Autodesk Inventor part; units mm, degrees
(part 13 of 16)
  spline S79 degree 3 poles (53.7291, 72.5452) (53.576, 72.5257) (53.422, 72.5132) (53.2678, 72.5092) (53.222, 72.508) (53.1761, 72.5076) (53.1303, 72.5079) (53.0872, 72.5083) (53.0441, 72.5093) (53.001, 72.5111) (52.9608, 72.5127) (52.9205, 72.515) (52.8803, 72.518) (52.8429, 72.5208) (52.8055, 72.5243) (52.7682, 72.5283) (52.7337, 72.5321) (52.6992, 72.5364) (52.6648, 72.5413) (52.6332, 72.5458) (52.6016, 72.5509) (52.5701, 72.5565) (52.5414, 72.5616) (52.5127, 72.5671) (52.4842, 72.5732) (52.4584, 72.5787) (52.4327, 72.5846) (52.407, 72.5909) (52.384, 72.5965) (52.3611, 72.6024) (52.3385, 72.6091) (52.3186, 72.615) (52.2989, 72.6215) (52.2786, 72.6272) (52.2408, 72.6377) (52.2006, 72.6455) (52.1693, 72.667) (52.1455, 72.6832) (52.1269, 72.7073) (52.1064, 72.7287) (52.0892, 72.7466) (52.0706, 72.7625) (52.0521, 72.7786) (52.034, 72.7943) (52.016, 72.8102) (51.9977, 72.8256) (51.9798, 72.8407) (51.9617, 72.8554) (51.9433, 72.8698) (51.9254, 72.8839) (51.9073, 72.8977) (51.889, 72.9112) (51.8711, 72.9244) (51.8531, 72.9372) (51.8348, 72.9498) (51.8169, 72.962) (51.7989, 72.974) (51.7806, 72.9856) (51.7628, 72.9969) (51.7448, 73.0079) (51.7266, 73.0186) (51.7088, 73.029) (51.6909, 73.0391) (51.6727, 73.0489) (51.655, 73.0584) (51.6371, 73.0676) (51.619, 73.0764) (51.6013, 73.085) (51.5834, 73.0933) (51.5653, 73.1012) (51.5476, 73.1089) (51.5298, 73.1162) (51.5118, 73.1232) (51.4941, 73.13) (51.4762, 73.1364) (51.4582, 73.1424) (51.4405, 73.1483) (51.4226, 73.1538) (51.4046, 73.1588) (51.3868, 73.1638) (51.3689, 73.1683) (51.3509, 73.1724) (51.333, 73.1763) (51.315, 73.1799) (51.297, 73.1828) (51.2789, 73.1858) (51.2608, 73.1882) (51.2427, 73.1901) (51.2244, 73.192) (51.2062, 73.1933) (51.1879, 73.194) (51.1694, 73.1947) (51.151, 73.1947) (51.1325, 73.1941) (51.1138, 73.1935) (51.0951, 73.1922) (51.0765, 73.1901) (51.0575, 73.188) (51.0386, 73.1851) (51.0198, 73.1815) (51.0005, 73.1777) (50.9814, 73.173) (50.9626, 73.1675) (50.9431, 73.1618) (50.924, 73.1552) (50.9052, 73.1477) (50.8858, 73.1398) (50.8667, 73.131) (50.8483, 73.1211) (50.8291, 73.111) (50.8106, 73.0997) (50.7928, 73.0874) (50.7744, 73.0748) (50.7567, 73.061) (50.74, 73.0462) (50.7229, 73.0311) (50.7068, 73.0148) (50.6916, 72.9977) (50.6808, 72.9856) (50.6705, 72.973) (50.6603, 72.9603) (50.6116, 72.8993) (50.5669, 72.8352) (50.5184, 72.7741) (50.4699, 72.713) (50.4176, 72.6548) (50.3693, 72.5935) (50.3592, 72.5808) (50.3493, 72.5679) (50.3399, 72.5546) (50.3267, 72.5359) (50.3146, 72.5165) (50.3037, 72.4964) (50.2931, 72.4768) (50.2837, 72.4565) (50.2755, 72.4357) (50.2676, 72.4155) (50.2609, 72.3949) (50.2553, 72.374) (50.2499, 72.3538) (50.2456, 72.3332) (50.2424, 72.3125) (50.2393, 72.2925) (50.2372, 72.2724) (50.2361, 72.2521) (50.235, 72.2325) (50.2348, 72.2129) (50.2355, 72.1933) (50.2362, 72.1741) (50.2377, 72.1551) (50.24, 72.1361) (50.2422, 72.1175) (50.2451, 72.099) (50.2488, 72.0806) (50.2524, 72.0625) (50.2566, 72.0445) (50.2615, 72.0267) (50.2663, 72.0091) (50.2717, 71.9916) (50.2777, 71.9742) (50.2836, 71.957) (50.2901, 71.9399) (50.2971, 71.923) (50.3041, 71.9061) (50.3116, 71.8894) (50.3196, 71.8729) (50.3276, 71.8562) (50.336, 71.8398) (50.3449, 71.8236) (50.3539, 71.8072) (50.3633, 71.7911) (50.3731, 71.7751) (50.383, 71.759) (50.3933, 71.7431) (50.404, 71.7274) (50.4148, 71.7114) (50.426, 71.6957) (50.4376, 71.6802) (50.4494, 71.6644) (50.4615, 71.6489) (50.4739, 71.6336) (50.4866, 71.618) (50.4996, 71.6026) (50.5129, 71.5875) (50.5265, 71.572) (50.5404, 71.5568) (50.5546, 71.5419) (50.5692, 71.5266) (50.584, 71.5115) (50.5991, 71.4968) (50.6145, 71.4816) (50.6302, 71.4668) (50.6462, 71.4522) (50.6626, 71.4372) (50.6792, 71.4225) (50.6961, 71.4081) (50.7134, 71.3933) (50.7309, 71.3788) (50.7487, 71.3646) (50.7669, 71.35) (50.7854, 71.3357) (50.8041, 71.3217) (50.8233, 71.3074) (50.8429, 71.2935) (50.8623, 71.2794) (50.8821, 71.2651) (50.9019, 71.2506) (50.9232, 71.2379) (50.9486, 71.2227) (50.9764, 71.2101) (50.9976, 71.1907) (51.0256, 71.165) (51.0423, 71.1276) (51.0612, 71.0932) (51.0713, 71.0747) (51.0821, 71.0571) (51.0924, 71.039) (51.104, 71.0185) (51.1149, 70.9975) (51.1256, 70.9764) (51.1376, 70.9528) (51.1492, 70.9291) (51.1604, 70.9052) (51.1728, 70.8788) (51.1847, 70.8522) (51.1962, 70.8253) (51.2088, 70.796) (51.2209, 70.7664) (51.2325, 70.7366) (51.2451, 70.7042) (51.2571, 70.6716) (51.2686, 70.6388) (51.2811, 70.6034) (51.2929, 70.5678) (51.3041, 70.532) (51.3162, 70.4935) (51.3275, 70.4548) (51.3383, 70.416) (51.3498, 70.3745) (51.3606, 70.3328) (51.3707, 70.2909) (51.3814, 70.2463) (51.3914, 70.2015) (51.4007, 70.1566) (51.4318, 70.0055) (51.4546, 69.8527) (51.4704, 69.6993) knots 0 0 0 0 0.065113 0.065113 0.065113 0.084473 0.084473 0.084473 0.102659 0.102659 0.102659 0.119672 0.119672 0.119672 0.135512 0.135512 0.135512 0.150178 0.150178 0.150178 0.163672 0.163672 0.163672 0.175991 0.175991 0.175991 0.187138 0.187138 0.187138 0.197111 0.197111 0.197111 0.205911 0.205911 0.205911 0.222284 0.222284 0.222284 0.234681 0.234681 0.234681 0.24506 0.24506 0.24506 0.255176 0.255176 0.255176 0.265035 0.265035 0.265035 0.274643 0.274643 0.274643 0.284008 0.284008 0.284008 0.293139 0.293139 0.293139 0.302047 0.302047 0.302047 0.310743 0.310743 0.310743 0.319241 0.319241 0.319241 0.327556 0.327556 0.327556 0.335706 0.335706 0.335706 0.343713 0.343713 0.343713 0.351599 0.351599 0.351599 0.359392 0.359392 0.359392 0.367126 0.367126 0.367126 0.374835 0.374835 0.374835 0.382562 0.382562 0.382562 0.390352 0.390352 0.390352 0.398256 0.398256 0.398256 0.406325 0.406325 0.406325 0.41461 0.41461 0.41461 0.423156 0.423156 0.423156 0.431994 0.431994 0.431994 0.441132 0.441132 0.441132 0.450548 0.450548 0.450548 0.460189 0.460189 0.460189 0.467051 0.467051 0.467051 0.5 0.5 0.5 0.532949 0.532949 0.532949 0.539811 0.539811 0.539811 0.549452 0.549452 0.549452 0.558868 0.558868 0.558868 0.568006 0.568006 0.568006 0.576844 0.576844 0.576844 0.58539 0.58539 0.58539 0.593675 0.593675 0.593675 0.601744 0.601744 0.601744 0.609648 0.609648 0.609648 0.617438 0.617438 0.617438 0.625165 0.625165 0.625165 0.632874 0.632874 0.632874 0.640608 0.640608 0.640608 0.648401 0.648401 0.648401 0.656287 0.656287 0.656287 0.664294 0.664294 0.664294 0.672444 0.672444 0.672444 0.680759 0.680759 0.680759 0.689257 0.689257 0.689257 0.697953 0.697953 0.697953 0.706861 0.706861 0.706861 0.715992 0.715992 0.715992 0.725357 0.725357 0.725357 0.734965 0.734965 0.734965 0.744824 0.744824 0.744824 0.75494 0.75494 0.75494 0.765319 0.765319 0.765319 0.777716 0.777716 0.777716 0.794089 0.794089 0.794089 0.802889 0.802889 0.802889 0.812862 0.812862 0.812862 0.824009 0.824009 0.824009 0.836328 0.836328 0.836328 0.849822 0.849822 0.849822 0.864488 0.864488 0.864488 0.880328 0.880328 0.880328 0.897341 0.897341 0.897341 0.915527 0.915527 0.915527 0.934887 0.934887 0.934887 1 1 1 1
  arc A282 (53.7291, 72.5452) -> (54.1249, 73.4583) centre (45.7832, 76.5321) ccw
  spline S80 degree 3 poles (54.658, 77.0523) (54.5352, 76.9589) (54.4081, 76.8711) (54.2766, 76.7905) (54.2374, 76.7665) (54.1979, 76.7432) (54.1581, 76.7206) (54.1206, 76.6993) (54.0828, 76.6787) (54.0446, 76.6587) (54.0089, 76.64) (53.9729, 76.6219) (53.9366, 76.6044) (53.9027, 76.5881) (53.8687, 76.5724) (53.8343, 76.5572) (53.8025, 76.5432) (53.7705, 76.5297) (53.7383, 76.5168) (53.7086, 76.5049) (53.6787, 76.4935) (53.6487, 76.4826) (53.6213, 76.4726) (53.5937, 76.4631) (53.5659, 76.4541) (53.5408, 76.4459) (53.5156, 76.4382) (53.4902, 76.4308) (53.4675, 76.4242) (53.4446, 76.4178) (53.4218, 76.4123) (53.4016, 76.4075) (53.3813, 76.4033) (53.3609, 76.398) (53.3228, 76.3883) (53.2841, 76.3749) (53.2463, 76.3778) (53.2176, 76.3801) (53.1894, 76.3916) (53.161, 76.3998) (53.1371, 76.4067) (53.1131, 76.4112) (53.089, 76.4159) (53.0655, 76.4205) (53.042, 76.4252) (53.0184, 76.4295) (52.9954, 76.4336) (52.9723, 76.4372) (52.9492, 76.4406) (52.9267, 76.4438) (52.9041, 76.4467) (52.8815, 76.4492) (52.8594, 76.4517) (52.8373, 76.4538) (52.8152, 76.4555) (52.7936, 76.4572) (52.772, 76.4585) (52.7504, 76.4594) (52.7293, 76.4603) (52.7082, 76.4609) (52.6871, 76.461) (52.6665, 76.4612) (52.6459, 76.4609) (52.6253, 76.4603) (52.6052, 76.4597) (52.5851, 76.4587) (52.565, 76.4573) (52.5454, 76.4559) (52.5257, 76.4541) (52.5062, 76.4519) (52.487, 76.4497) (52.4678, 76.4472) (52.4488, 76.4442) (52.43, 76.4412) (52.4113, 76.4379) (52.3928, 76.4341) (52.3745, 76.4303) (52.3562, 76.4261) (52.3382, 76.4215) (52.3203, 76.4169) (52.3025, 76.4119) (52.2849, 76.4063) (52.2674, 76.4008) (52.2501, 76.3949) (52.2329, 76.3884) (52.2158, 76.382) (52.1989, 76.375) (52.1822, 76.3676) (52.1655, 76.3601) (52.1491, 76.3521) (52.1329, 76.3435) (52.1166, 76.3349) (52.1005, 76.3257) (52.0849, 76.316) (52.069, 76.3061) (52.0534, 76.2956) (52.0383, 76.2845) (52.0229, 76.2732) (52.008, 76.2612) (51.9936, 76.2487) (51.9788, 76.2357) (51.9646, 76.2222) (51.951, 76.208) (51.937, 76.1933) (51.9237, 76.178) (51.9112, 76.1621) (51.8983, 76.1456) (51.8863, 76.1284) (51.8752, 76.1106) (51.8637, 76.0923) (51.8533, 76.0733) (51.844, 76.0537) (51.8344, 76.0335) (51.826, 76.0128) (51.8189, 75.9916) (51.8117, 75.97) (51.8058, 75.9478) (51.8012, 75.9254) (51.798, 75.9095) (51.7953, 75.8935) (51.7929, 75.8774) (51.7811, 75.8002) (51.7744, 75.7223) (51.763, 75.6451) (51.7515, 75.568) (51.7354, 75.4915) (51.7242, 75.4142) (51.7218, 75.3981) (51.7197, 75.382) (51.7182, 75.3658) (51.7161, 75.3431) (51.7153, 75.3202) (51.7159, 75.2973) (51.7165, 75.275) (51.7186, 75.2528) (51.7219, 75.2307) (51.7251, 75.2093) (51.7296, 75.188) (51.7352, 75.1671) (51.7407, 75.1469) (51.7472, 75.127) (51.7548, 75.1074) (51.7621, 75.0886) (51.7704, 75.07) (51.7795, 75.052) (51.7884, 75.0345) (51.7981, 75.0173) (51.8085, 75.0007) (51.8186, 74.9845) (51.8294, 74.9687) (51.8409, 74.9534) (51.8521, 74.9384) (51.8639, 74.9239) (51.8763, 74.9098) (51.8884, 74.8959) (51.9011, 74.8825) (51.9142, 74.8695) (51.9272, 74.8566) (51.9407, 74.8441) (51.9545, 74.8321) (51.9683, 74.8201) (51.9824, 74.8086) (51.9969, 74.7975) (52.0115, 74.7863) (52.0263, 74.7756) (52.0415, 74.7653) (52.0567, 74.7549) (52.0723, 74.7449) (52.088, 74.7353) (52.104, 74.7256) (52.1202, 74.7163) (52.1366, 74.7074) (52.1533, 74.6983) (52.1702, 74.6897) (52.1873, 74.6815) (52.2047, 74.6731) (52.2223, 74.6651) (52.24, 74.6574) (52.2581, 74.6496) (52.2763, 74.6422) (52.2947, 74.6352) (52.3136, 74.628) (52.3325, 74.6212) (52.3516, 74.6148) (52.3711, 74.6082) (52.3908, 74.602) (52.4105, 74.5962) (52.4307, 74.5902) (52.4511, 74.5846) (52.4715, 74.5793) (52.4925, 74.5739) (52.5135, 74.5689) (52.5347, 74.5643) (52.5563, 74.5595) (52.5781, 74.5551) (52.5999, 74.551) (52.6223, 74.5469) (52.6447, 74.5431) (52.6672, 74.5397) (52.6903, 74.5361) (52.7134, 74.5329) (52.7366, 74.5302) (52.7605, 74.5274) (52.7843, 74.5251) (52.8081, 74.5227) (52.8326, 74.5202) (52.8569, 74.5175) (52.8817, 74.5172) (52.9113, 74.5167) (52.9417, 74.5196) (52.9697, 74.5135) (53.0068, 74.5053) (53.04, 74.4812) (53.0735, 74.4609) (53.0916, 74.4499) (53.1097, 74.44) (53.1276, 74.4295) (53.1479, 74.4176) (53.1679, 74.4049) (53.1877, 74.3919) (53.2099, 74.3775) (53.2318, 74.3628) (53.2535, 74.3477) (53.2774, 74.331) (53.3011, 74.3139) (53.3244, 74.2964) (53.35, 74.2773) (53.3753, 74.2577) (53.4002, 74.2377) (53.4273, 74.2159) (53.454, 74.1937) (53.4804, 74.1711) (53.5089, 74.1466) (53.5369, 74.1217) (53.5645, 74.0963) (53.5942, 74.069) (53.6234, 74.0412) (53.6521, 74.0129) (53.6829, 73.9827) (53.7131, 73.952) (53.7427, 73.9208) (53.7744, 73.8875) (53.8054, 73.8538) (53.8359, 73.8195) (53.9383, 73.7042) (54.0345, 73.5833) (54.1249, 73.4583) knots 0 0 0 0 0.065113 0.065113 0.065113 0.084473 0.084473 0.084473 0.102659 0.102659 0.102659 0.119672 0.119672 0.119672 0.135512 0.135512 0.135512 0.150178 0.150178 0.150178 0.163672 0.163672 0.163672 0.175991 0.175991 0.175991 0.187138 0.187138 0.187138 0.197111 0.197111 0.197111 0.205911 0.205911 0.205911 0.222284 0.222284 0.222284 0.234681 0.234681 0.234681 0.24506 0.24506 0.24506 0.255176 0.255176 0.255176 0.265035 0.265035 0.265035 0.274643 0.274643 0.274643 0.284008 0.284008 0.284008 0.293139 0.293139 0.293139 0.302047 0.302047 0.302047 0.310743 0.310743 0.310743 0.319241 0.319241 0.319241 0.327556 0.327556 0.327556 0.335706 0.335706 0.335706 0.343713 0.343713 0.343713 0.351599 0.351599 0.351599 0.359392 0.359392 0.359392 0.367126 0.367126 0.367126 0.374835 0.374835 0.374835 0.382562 0.382562 0.382562 0.390352 0.390352 0.390352 0.398256 0.398256 0.398256 0.406325 0.406325 0.406325 0.41461 0.41461 0.41461 0.423156 0.423156 0.423156 0.431994 0.431994 0.431994 0.441132 0.441132 0.441132 0.450548 0.450548 0.450548 0.460189 0.460189 0.460189 0.467051 0.467051 0.467051 0.5 0.5 0.5 0.532949 0.532949 0.532949 0.539811 0.539811 0.539811 0.549452 0.549452 0.549452 0.558868 0.558868 0.558868 0.568006 0.568006 0.568006 0.576844 0.576844 0.576844 0.58539 0.58539 0.58539 0.593675 0.593675 0.593675 0.601744 0.601744 0.601744 0.609648 0.609648 0.609648 0.617438 0.617438 0.617438 0.625165 0.625165 0.625165 0.632874 0.632874 0.632874 0.640608 0.640608 0.640608 0.648401 0.648401 0.648401 0.656287 0.656287 0.656287 0.664294 0.664294 0.664294 0.672444 0.672444 0.672444 0.680759 0.680759 0.680759 0.689257 0.689257 0.689257 0.697953 0.697953 0.697953 0.706861 0.706861 0.706861 0.715992 0.715992 0.715992 0.725357 0.725357 0.725357 0.734965 0.734965 0.734965 0.744824 0.744824 0.744824 0.75494 0.75494 0.75494 0.765319 0.765319 0.765319 0.777716 0.777716 0.777716 0.794089 0.794089 0.794089 0.802889 0.802889 0.802889 0.812862 0.812862 0.812862 0.824009 0.824009 0.824009 0.836328 0.836328 0.836328 0.849822 0.849822 0.849822 0.864488 0.864488 0.864488 0.880328 0.880328 0.880328 0.897341 0.897341 0.897341 0.915527 0.915527 0.915527 0.934887 0.934887 0.934887 1 1 1 1
  arc A283 (54.658, 77.0523) -> (54.5443, 78.0409) centre (45.7832, 76.5321) ccw
  spline S81 degree 3 poles (53.2089, 81.42) (53.1493, 81.2777) (53.0831, 81.1381) (53.0095, 81.0026) (52.9876, 80.9623) (52.965, 80.9223) (52.9418, 80.8828) (52.92, 80.8456) (52.8976, 80.8088) (52.8745, 80.7724) (52.8529, 80.7384) (52.8308, 80.7047) (52.8081, 80.6714) (52.787, 80.6404) (52.7653, 80.6097) (52.7431, 80.5794) (52.7226, 80.5514) (52.7016, 80.5237) (52.6802, 80.4964) (52.6604, 80.4712) (52.6403, 80.4464) (52.6197, 80.4219) (52.6009, 80.3996) (52.5818, 80.3775) (52.5623, 80.3559) (52.5446, 80.3363) (52.5266, 80.317) (52.5083, 80.2979) (52.4919, 80.2808) (52.4754, 80.2639) (52.4583, 80.2476) (52.4432, 80.2333) (52.4278, 80.2196) (52.4127, 80.2048) (52.3847, 80.1774) (52.3578, 80.1464) (52.3236, 80.13) (52.2976, 80.1176) (52.2675, 80.1136) (52.2387, 80.1064) (52.2146, 80.1005) (52.1915, 80.0923) (52.1683, 80.0843) (52.1457, 80.0766) (52.1229, 80.0689) (52.1004, 80.0608) (52.0784, 80.0529) (52.0566, 80.0445) (52.0349, 80.0358) (52.0138, 80.0273) (51.9928, 80.0186) (51.9719, 80.0094) (51.9516, 80.0006) (51.9314, 79.9913) (51.9114, 79.9818) (51.8919, 79.9724) (51.8725, 79.9628) (51.8534, 79.9528) (51.8346, 79.943) (51.8161, 79.9329) (51.7977, 79.9225) (51.7798, 79.9123) (51.7621, 79.9018) (51.7446, 79.891) (51.7275, 79.8804) (51.7106, 79.8695) (51.6939, 79.8582) (51.6776, 79.8472) (51.6614, 79.8358) (51.6456, 79.8241) (51.6301, 79.8127) (51.6148, 79.8009) (51.5997, 79.7887) (51.585, 79.7768) (51.5705, 79.7646) (51.5563, 79.752) (51.5423, 79.7396) (51.5286, 79.7269) (51.5153, 79.7138) (51.5021, 79.7009) (51.4892, 79.6876) (51.4767, 79.674) (51.4643, 79.6605) (51.4523, 79.6467) (51.4407, 79.6325) (51.4291, 79.6184) (51.4179, 79.6039) (51.4072, 79.5891) (51.3965, 79.5743) (51.3862, 79.5591) (51.3765, 79.5436) (51.3667, 79.528) (51.3574, 79.512) (51.3487, 79.4958) (51.3399, 79.4792) (51.3317, 79.4624) (51.3241, 79.4452) (51.3165, 79.4277) (51.3095, 79.4099) (51.3033, 79.3918) (51.2969, 79.3732) (51.2914, 79.3544) (51.2867, 79.3353) (51.2819, 79.3156) (51.2781, 79.2957) (51.2753, 79.2757) (51.2723, 79.2549) (51.2705, 79.234) (51.2698, 79.2131) (51.269, 79.1914) (51.2695, 79.1698) (51.2712, 79.1482) (51.273, 79.1259) (51.2761, 79.1038) (51.2805, 79.0819) (51.2851, 79.0595) (51.2911, 79.0374) (51.2983, 79.0157) (51.3034, 79.0003) (51.3092, 78.9851) (51.3151, 78.9699) (51.3435, 78.8972) (51.3767, 78.8264) (51.4054, 78.7539) (51.434, 78.6813) (51.4582, 78.607) (51.4872, 78.5345) (51.4932, 78.5194) (51.4994, 78.5043) (51.5062, 78.4896) (51.5158, 78.4688) (51.5265, 78.4486) (51.5385, 78.4291) (51.5502, 78.4101) (51.5631, 78.3918) (51.577, 78.3744) (51.5905, 78.3575) (51.605, 78.3413) (51.6203, 78.326) (51.6351, 78.3112) (51.6508, 78.2972) (51.6671, 78.2841) (51.6829, 78.2714) (51.6993, 78.2595) (51.7162, 78.2484) (51.7327, 78.2377) (51.7496, 78.2277) (51.767, 78.2185) (51.7838, 78.2095) (51.8011, 78.2013) (51.8187, 78.1938) (51.8359, 78.1864) (51.8534, 78.1797) (51.8711, 78.1737) (51.8886, 78.1677) (51.9063, 78.1624) (51.9242, 78.1577) (51.9419, 78.1531) (51.9597, 78.149) (51.9777, 78.1455) (51.9956, 78.142) (52.0137, 78.1391) (52.0318, 78.1367) (52.0499, 78.1343) (52.0682, 78.1325) (52.0865, 78.1311) (52.1049, 78.1297) (52.1233, 78.1288) (52.1418, 78.1284) (52.1605, 78.128) (52.1791, 78.1281) (52.1978, 78.1286) (52.2168, 78.1291) (52.2357, 78.1301) (52.2547, 78.1314) (52.2739, 78.1329) (52.2931, 78.1347) (52.3123, 78.137) (52.3319, 78.1393) (52.3514, 78.142) (52.3708, 78.1451) (52.3907, 78.1483) (52.4105, 78.1519) (52.4303, 78.1558) (52.4505, 78.1599) (52.4706, 78.1644) (52.4906, 78.1692) (52.5111, 78.1741) (52.5316, 78.1794) (52.5519, 78.1851) (52.5727, 78.1909) (52.5935, 78.1971) (52.6141, 78.2036) (52.6352, 78.2103) (52.6563, 78.2174) (52.6772, 78.2248) (52.6986, 78.2324) (52.72, 78.2404) (52.7412, 78.2486) (52.7629, 78.2571) (52.7846, 78.2659) (52.806, 78.2751) (52.8281, 78.2846) (52.8499, 78.2946) (52.8717, 78.3044) (52.8941, 78.3144) (52.9165, 78.3243) (52.9382, 78.3364) (52.9641, 78.3508) (52.9889, 78.3685) (53.0163, 78.3772) (53.0525, 78.3886) (53.0932, 78.3844) (53.1325, 78.3835) (53.1535, 78.3831) (53.1742, 78.3836) (53.195, 78.3834) (53.2185, 78.3832) (53.2422, 78.3822) (53.2658, 78.3809) (53.2922, 78.3795) (53.3186, 78.3777) (53.3449, 78.3755) (53.3739, 78.373) (53.403, 78.37) (53.432, 78.3666) (53.4637, 78.3628) (53.4954, 78.3584) (53.527, 78.3536) (53.5613, 78.3483) (53.5956, 78.3424) (53.6297, 78.336) (53.6666, 78.329) (53.7033, 78.3214) (53.74, 78.3133) (53.7793, 78.3045) (53.8185, 78.295) (53.8575, 78.2849) (53.8992, 78.2741) (53.9407, 78.2626) (53.9821, 78.2504) (54.026, 78.2374) (54.0698, 78.2237) (54.1133, 78.2092) (54.2597, 78.1606) (54.4035, 78.104) (54.5443, 78.0409) knots 0 0 0 0 0.065113 0.065113 0.065113 0.084473 0.084473 0.084473 0.102659 0.102659 0.102659 0.119672 0.119672 0.119672 0.135512 0.135512 0.135512 0.150178 0.150178 0.150178 0.163672 0.163672 0.163672 0.175991 0.175991 0.175991 0.187138 0.187138 0.187138 0.197111 0.197111 0.197111 0.205911 0.205911 0.205911 0.222284 0.222284 0.222284 0.234681 0.234681 0.234681 0.24506 0.24506 0.24506 0.255176 0.255176 0.255176 0.265035 0.265035 0.265035 0.274643 0.274643 0.274643 0.284008 0.284008 0.284008 0.293139 0.293139 0.293139 0.302047 0.302047 0.302047 0.310743 0.310743 0.310743 0.319241 0.319241 0.319241 0.327556 0.327556 0.327556 0.335706 0.335706 0.335706 0.343713 0.343713 0.343713 0.351599 0.351599 0.351599 0.359392 0.359392 0.359392 0.367126 0.367126 0.367126 0.374835 0.374835 0.374835 0.382562 0.382562 0.382562 0.390352 0.390352 0.390352 0.398256 0.398256 0.398256 0.406325 0.406325 0.406325 0.41461 0.41461 0.41461 0.423156 0.423156 0.423156 0.431994 0.431994 0.431994 0.441132 0.441132 0.441132 0.450548 0.450548 0.450548 0.460189 0.460189 0.460189 0.467051 0.467051 0.467051 0.5 0.5 0.5 0.532949 0.532949 0.532949 0.539811 0.539811 0.539811 0.549452 0.549452 0.549452 0.558868 0.558868 0.558868 0.568006 0.568006 0.568006 0.576844 0.576844 0.576844 0.58539 0.58539 0.58539 0.593675 0.593675 0.593675 0.601744 0.601744 0.601744 0.609648 0.609648 0.609648 0.617438 0.617438 0.617438 0.625165 0.625165 0.625165 0.632874 0.632874 0.632874 0.640608 0.640608 0.640608 0.648401 0.648401 0.648401 0.656287 0.656287 0.656287 0.664294 0.664294 0.664294 0.672444 0.672444 0.672444 0.680759 0.680759 0.680759 0.689257 0.689257 0.689257 0.697953 0.697953 0.697953 0.706861 0.706861 0.706861 0.715992 0.715992 0.715992 0.725357 0.725357 0.725357 0.734965 0.734965 0.734965 0.744824 0.744824 0.744824 0.75494 0.75494 0.75494 0.765319 0.765319 0.765319 0.777716 0.777716 0.777716 0.794089 0.794089 0.794089 0.802889 0.802889 0.802889 0.812862 0.812862 0.812862 0.824009 0.824009 0.824009 0.836328 0.836328 0.836328 0.849822 0.849822 0.849822 0.864488 0.864488 0.864488 0.880328 0.880328 0.880328 0.897341 0.897341 0.897341 0.915527 0.915527 0.915527 0.934887 0.934887 0.934887 1 1 1 1
  arc A284 (53.2089, 81.42) -> (52.6161, 82.2193) centre (45.7832, 76.5321) ccw
  spline S82 degree 3 poles (49.7702, 84.478) (49.7897, 84.3249) (49.8021, 84.171) (49.8061, 84.0168) (49.8073, 83.9709) (49.8078, 83.925) (49.8074, 83.8792) (49.8071, 83.8361) (49.8061, 83.793) (49.8043, 83.75) (49.8026, 83.7097) (49.8003, 83.6695) (49.7973, 83.6293) (49.7945, 83.5918) (49.7911, 83.5545) (49.787, 83.5172) (49.7833, 83.4826) (49.779, 83.4481) (49.774, 83.4137) (49.7695, 83.3821) (49.7645, 83.3505) (49.7589, 83.3191) (49.7538, 83.2903) (49.7483, 83.2616) (49.7422, 83.2331) (49.7367, 83.2073) (49.7307, 83.1816) (49.7244, 83.1559) (49.7188, 83.1329) (49.7129, 83.11) (49.7063, 83.0874) (49.7004, 83.0675) (49.6939, 83.0478) (49.6882, 83.0275) (49.6776, 82.9897) (49.6699, 82.9495) (49.6484, 82.9182) (49.6321, 82.8945) (49.608, 82.8759) (49.5867, 82.8553) (49.5688, 82.8381) (49.5529, 82.8195) (49.5368, 82.801) (49.5211, 82.7829) (49.5052, 82.7649) (49.4897, 82.7466) (49.4746, 82.7288) (49.46, 82.7106) (49.4455, 82.6923) (49.4315, 82.6744) (49.4177, 82.6563) (49.4042, 82.6379) (49.391, 82.6201) (49.3781, 82.602) (49.3656, 82.5837) (49.3533, 82.5659) (49.3414, 82.5478) (49.3298, 82.5296) (49.3185, 82.5118) (49.3075, 82.4937) (49.2968, 82.4755) (49.2864, 82.4578) (49.2763, 82.4398) (49.2665, 82.4217) (49.257, 82.4039) (49.2478, 82.386) (49.239, 82.3679) (49.2304, 82.3502) (49.2221, 82.3323) (49.2142, 82.3143) (49.2065, 82.2966) (49.1991, 82.2787) (49.1922, 82.2607) (49.1853, 82.243) (49.1789, 82.2251) (49.1729, 82.2071) (49.167, 82.1894) (49.1615, 82.1716) (49.1565, 82.1536) (49.1516, 82.1358) (49.147, 82.1179) (49.143, 82.0998) (49.139, 82.082) (49.1355, 82.064) (49.1325, 82.0459) (49.1296, 82.0279) (49.1271, 82.0098) (49.1252, 81.9916) (49.1234, 81.9734) (49.1221, 81.9551) (49.1214, 81.9368) (49.1207, 81.9184) (49.1206, 81.8999) (49.1212, 81.8814) (49.1219, 81.8627) (49.1232, 81.844) (49.1253, 81.8254) (49.1274, 81.8064) (49.1302, 81.7875) (49.1339, 81.7687) (49.1377, 81.7495) (49.1423, 81.7304) (49.1478, 81.7115) (49.1535, 81.6921) (49.1601, 81.6729) (49.1677, 81.6541) (49.1755, 81.6347) (49.1844, 81.6157) (49.1942, 81.5972) (49.2044, 81.5781) (49.2157, 81.5595) (49.2279, 81.5417) (49.2406, 81.5233) (49.2544, 81.5057) (49.2692, 81.489) (49.2843, 81.4718) (49.3006, 81.4557) (49.3176, 81.4405) (49.3298, 81.4297) (49.3424, 81.4194) (49.3551, 81.4093) (49.416, 81.3605) (49.4801, 81.3158) (49.5413, 81.2673) (49.6024, 81.2188) (49.6605, 81.1665) (49.7218, 81.1182) (49.7346, 81.1081) (49.7475, 81.0982) (49.7608, 81.0888) (49.7794, 81.0757) (49.7988, 81.0635) (49.8189, 81.0526) (49.8386, 81.042) (49.8589, 81.0326) (49.8797, 81.0245) (49.8998, 81.0166) (49.9204, 81.0098) (49.9414, 81.0042) (49.9616, 80.9988) (49.9821, 80.9945) (50.0028, 80.9913) (50.0228, 80.9882) (50.043, 80.9861) (50.0632, 80.985) (50.0828, 80.9839) (50.1025, 80.9837) (50.1221, 80.9844) (50.1412, 80.9851) (50.1603, 80.9866) (50.1793, 80.9889) (50.1979, 80.9911) (50.2164, 80.9941) (50.2348, 80.9977) (50.2529, 81.0013) (50.2708, 81.0055) (50.2886, 81.0104) (50.3063, 81.0152) (50.3238, 81.0206) (50.3411, 81.0266) (50.3584, 81.0326) (50.3755, 81.039) (50.3923, 81.046) (50.4093, 81.053) (50.426, 81.0605) (50.4425, 81.0685) (50.4591, 81.0765) (50.4756, 81.085) (50.4918, 81.0938) (50.5081, 81.1028) (50.5243, 81.1122) (50.5402, 81.122) (50.5564, 81.1319) (50.5723, 81.1422) (50.588, 81.1529) (50.604, 81.1637) (50.6197, 81.175) (50.6352, 81.1865) (50.651, 81.1983) (50.6665, 81.2104) (50.6818, 81.2228) (50.6974, 81.2355) (50.7128, 81.2485) (50.7279, 81.2618) (50.7433, 81.2755) (50.7585, 81.2894) (50.7735, 81.3036) (50.7888, 81.3181) (50.8038, 81.3329) (50.8186, 81.348) (50.8337, 81.3634) (50.8486, 81.3792) (50.8632, 81.3951) (50.8782, 81.4115) (50.8928, 81.4281) (50.9072, 81.445) (50.922, 81.4623) (50.9365, 81.4799) (50.9508, 81.4976) (50.9654, 81.5159) (50.9797, 81.5343) (50.9937, 81.553) (51.008, 81.5722) (51.0219, 81.5918) (51.0359, 81.6112) (51.0503, 81.6311) (51.0648, 81.6508) (51.0775, 81.6721) (51.0927, 81.6976) (51.1053, 81.7253) (51.1247, 81.7465) (51.1503, 81.7745) (51.1877, 81.7912) (51.2222, 81.8101) (51.2407, 81.8202) (51.2583, 81.831) (51.2764, 81.8413) (51.2968, 81.8529) (51.3179, 81.8639) (51.339, 81.8745) (51.3625, 81.8865) (51.3862, 81.8981) (51.4101, 81.9093) (51.4365, 81.9218) (51.4632, 81.9337) (51.49, 81.9452) (51.5194, 81.9577) (51.549, 81.9698) (51.5788, 81.9814) (51.6112, 81.994) (51.6438, 82.006) (51.6766, 82.0175) (51.712, 82.03) (51.7476, 82.0418) (51.7834, 82.053) (51.8219, 82.0651) (51.8605, 82.0765) (51.8994, 82.0872) (51.9409, 82.0987) (51.9826, 82.1095) (52.0245, 82.1196) (52.0691, 82.1304) (52.1139, 82.1403) (52.1588, 82.1496) (52.3099, 82.1807) (52.4626, 82.2035) (52.6161, 82.2193) knots 0 0 0 0 0.065113 0.065113 0.065113 0.084473 0.084473 0.084473 0.102659 0.102659 0.102659 0.119672 0.119672 0.119672 0.135512 0.135512 0.135512 0.150178 0.150178 0.150178 0.163672 0.163672 0.163672 0.175991 0.175991 0.175991 0.187138 0.187138 0.187138 0.197111 0.197111 0.197111 0.205911 0.205911 0.205911 0.222284 0.222284 0.222284 0.234681 0.234681 0.234681 0.24506 0.24506 0.24506 0.255176 0.255176 0.255176 0.265035 0.265035 0.265035 0.274643 0.274643 0.274643 0.284008 0.284008 0.284008 0.293139 0.293139 0.293139 0.302047 0.302047 0.302047 0.310743 0.310743 0.310743 0.319241 0.319241 0.319241 0.327556 0.327556 0.327556 0.335706 0.335706 0.335706 0.343713 0.343713 0.343713 0.351599 0.351599 0.351599 0.359392 0.359392 0.359392 0.367126 0.367126 0.367126 0.374835 0.374835 0.374835 0.382562 0.382562 0.382562 0.390352 0.390352 0.390352 0.398256 0.398256 0.398256 0.406325 0.406325 0.406325 0.41461 0.41461 0.41461 0.423156 0.423156 0.423156 0.431994 0.431994 0.431994 0.441132 0.441132 0.441132 0.450548 0.450548 0.450548 0.460189 0.460189 0.460189 0.467051 0.467051 0.467051 0.5 0.5 0.5 0.532949 0.532949 0.532949 0.539811 0.539811 0.539811 0.549452 0.549452 0.549452 0.558868 0.558868 0.558868 0.568006 0.568006 0.568006 0.576844 0.576844 0.576844 0.58539 0.58539 0.58539 0.593675 0.593675 0.593675 0.601744 0.601744 0.601744 0.609648 0.609648 0.609648 0.617438 0.617438 0.617438 0.625165 0.625165 0.625165 0.632874 0.632874 0.632874 0.640608 0.640608 0.640608 0.648401 0.648401 0.648401 0.656287 0.656287 0.656287 0.664294 0.664294 0.664294 0.672444 0.672444 0.672444 0.680759 0.680759 0.680759 0.689257 0.689257 0.689257 0.697953 0.697953 0.697953 0.706861 0.706861 0.706861 0.715992 0.715992 0.715992 0.725357 0.725357 0.725357 0.734965 0.734965 0.734965 0.744824 0.744824 0.744824 0.75494 0.75494 0.75494 0.765319 0.765319 0.765319 0.777716 0.777716 0.777716 0.794089 0.794089 0.794089 0.802889 0.802889 0.802889 0.812862 0.812862 0.812862 0.824009 0.824009 0.824009 0.836328 0.836328 0.836328 0.849822 0.849822 0.849822 0.864488 0.864488 0.864488 0.880328 0.880328 0.880328 0.897341 0.897341 0.897341 0.915527 0.915527 0.915527 0.934887 0.934887 0.934887 1 1 1 1
  arc A285 (49.7702, 84.478) -> (48.8571, 84.8738) centre (45.7832, 76.5321) ccw
  spline S83 degree 3 poles (45.2631, 85.4069) (45.3565, 85.2841) (45.4443, 85.157) (45.5249, 85.0255) (45.5488, 84.9864) (45.5721, 84.9469) (45.5948, 84.907) (45.616, 84.8695) (45.6367, 84.8317) (45.6567, 84.7935) (45.6754, 84.7578) (45.6935, 84.7218) (45.711, 84.6855) (45.7273, 84.6517) (45.743, 84.6176) (45.7581, 84.5833) (45.7721, 84.5515) (45.7856, 84.5194) (45.7986, 84.4872) (45.8105, 84.4575) (45.8219, 84.4277) (45.8328, 84.3976) (45.8428, 84.3702) (45.8523, 84.3426) (45.8613, 84.3148) (45.8694, 84.2897) (45.8771, 84.2645) (45.8845, 84.2391) (45.8912, 84.2164) (45.8975, 84.1936) (45.903, 84.1707) (45.9079, 84.1505) (45.9121, 84.1302) (45.9173, 84.1098) (45.9271, 84.0718) (45.9405, 84.0331) (45.9375, 83.9952) (45.9353, 83.9665) (45.9237, 83.9384) (45.9155, 83.9099) (45.9087, 83.886) (45.9042, 83.862) (45.8995, 83.8379) (45.8949, 83.8144) (45.8901, 83.7909) (45.8859, 83.7673) (45.8818, 83.7443) (45.8781, 83.7212) (45.8748, 83.6981) (45.8716, 83.6756) (45.8687, 83.653) (45.8661, 83.6304) (45.8637, 83.6083) (45.8616, 83.5862) (45.8599, 83.5641) (45.8582, 83.5426) (45.8569, 83.521) (45.8559, 83.4993) (45.855, 83.4783) (45.8545, 83.4572) (45.8543, 83.4361) (45.8542, 83.4155) (45.8544, 83.3949) (45.8551, 83.3743) (45.8557, 83.3541) (45.8567, 83.334) (45.8581, 83.3139) (45.8595, 83.2943) (45.8613, 83.2747) (45.8635, 83.2551) (45.8656, 83.2359) (45.8682, 83.2168) (45.8712, 83.1977) (45.8741, 83.1789) (45.8775, 83.1603) (45.8813, 83.1417) (45.885, 83.1234) (45.8892, 83.1052) (45.8939, 83.0871) (45.8985, 83.0692) (45.9035, 83.0514) (45.909, 83.0338) (45.9145, 83.0163) (45.9205, 82.999) (45.9269, 82.9818) (45.9334, 82.9647) (45.9403, 82.9478) (45.9478, 82.9312) (45.9553, 82.9145) (45.9633, 82.898) (45.9718, 82.8818) (45.9804, 82.8655) (45.9896, 82.8495) (45.9994, 82.8338) (46.0093, 82.8179) (46.0198, 82.8024) (46.0309, 82.7873) (46.0422, 82.7719) (46.0541, 82.7569) (46.0667, 82.7425) (46.0796, 82.7277) (46.0932, 82.7135) (46.1074, 82.6999) (46.122, 82.6859) (46.1373, 82.6726) (46.1533, 82.6601) (46.1698, 82.6472) (46.1869, 82.6352) (46.2047, 82.6241) (46.2231, 82.6126) (46.2421, 82.6022) (46.2617, 82.5929) (46.2818, 82.5833) (46.3026, 82.5749) (46.3237, 82.5678) (46.3454, 82.5606) (46.3675, 82.5548) (46.3899, 82.5502) (46.4058, 82.5469) (46.4219, 82.5442) (46.438, 82.5418) (46.5151, 82.5301) (46.593, 82.5234) (46.6702, 82.5119) (46.7474, 82.5005) (46.8239, 82.4843) (46.9011, 82.4731) (46.9172, 82.4707) (46.9333, 82.4686) (46.9495, 82.4671) (46.9723, 82.4651) (46.9952, 82.4642) (47.018, 82.4648) (47.0403, 82.4655) (47.0626, 82.4675) (47.0847, 82.4708) (47.1061, 82.4741) (47.1273, 82.4785) (47.1482, 82.4841) (47.1685, 82.4896) (47.1884, 82.4961) (47.2079, 82.5037) (47.2268, 82.511) (47.2453, 82.5193) (47.2634, 82.5284) (47.2809, 82.5373) (47.298, 82.547) (47.3147, 82.5574) (47.3309, 82.5675) (47.3466, 82.5784) (47.362, 82.5898) (47.377, 82.601) (47.3915, 82.6129) (47.4056, 82.6252) (47.4195, 82.6374) (47.4329, 82.65) (47.4459, 82.6631) (47.4588, 82.6761) (47.4712, 82.6896) (47.4832, 82.7034) (47.4952, 82.7172) (47.5068, 82.7314) (47.5179, 82.7458) (47.5291, 82.7604) (47.5398, 82.7752) (47.5501, 82.7904) (47.5605, 82.8056) (47.5705, 82.8212) (47.5801, 82.837) (47.5898, 82.8529) (47.5991, 82.8691) (47.608, 82.8856) (47.617, 82.9022) (47.6257, 82.9191) (47.6339, 82.9362) (47.6423, 82.9536) (47.6503, 82.9712) (47.6579, 82.9889) (47.6657, 83.007) (47.6731, 83.0253) (47.6802, 83.0437) (47.6873, 83.0625) (47.6941, 83.0814) (47.7006, 83.1005) (47.7072, 83.12) (47.7134, 83.1397) (47.7192, 83.1594) (47.7252, 83.1797) (47.7308, 83.2) (47.7361, 83.2205) (47.7414, 83.2414) (47.7465, 83.2625) (47.7511, 83.2836) (47.7559, 83.3053) (47.7603, 83.327) (47.7643, 83.3488) (47.7685, 83.3712) (47.7722, 83.3937) (47.7757, 83.4161) (47.7792, 83.4392) (47.7824, 83.4624) (47.7852, 83.4856) (47.788, 83.5094) (47.7902, 83.5333) (47.7927, 83.5571) (47.7952, 83.5815) (47.7979, 83.6058) (47.7982, 83.6306) (47.7986, 83.6603) (47.7957, 83.6906) (47.8019, 83.7187) (47.8101, 83.7557) (47.8341, 83.7889) (47.8545, 83.8225) (47.8654, 83.8405) (47.8753, 83.8587) (47.8859, 83.8766) (47.8978, 83.8969) (47.9105, 83.9169) (47.9234, 83.9367) (47.9379, 83.9588) (47.9526, 83.9807) (47.9677, 84.0024) (47.9843, 84.0263) (48.0015, 84.05) (48.0189, 84.0733) (48.0381, 84.0989) (48.0577, 84.1242) (48.0777, 84.1491) (48.0994, 84.1762) (48.1217, 84.203) (48.1443, 84.2293) (48.1688, 84.2578) (48.1937, 84.2858) (48.2191, 84.3134) (48.2464, 84.3431) (48.2742, 84.3723) (48.3024, 84.4011) (48.3326, 84.4318) (48.3634, 84.462) (48.3946, 84.4917) (48.4278, 84.5233) (48.4616, 84.5543) (48.4959, 84.5848) (48.6112, 84.6873) (48.7321, 84.7834) (48.8571, 84.8738) knots 0 0 0 0 0.065113 0.065113 0.065113 0.084473 0.084473 0.084473 0.102659 0.102659 0.102659 0.119672 0.119672 0.119672 0.135512 0.135512 0.135512 0.150178 0.150178 0.150178 0.163672 0.163672 0.163672 0.175991 0.175991 0.175991 0.187138 0.187138 0.187138 0.197111 0.197111 0.197111 0.205911 0.205911 0.205911 0.222284 0.222284 0.222284 0.234681 0.234681 0.234681 0.24506 0.24506 0.24506 0.255176 0.255176 0.255176 0.265035 0.265035 0.265035 0.274643 0.274643 0.274643 0.284008 0.284008 0.284008 0.293139 0.293139 0.293139 0.302047 0.302047 0.302047 0.310743 0.310743 0.310743 0.319241 0.319241 0.319241 0.327556 0.327556 0.327556 0.335706 0.335706 0.335706 0.343713 0.343713 0.343713 0.351599 0.351599 0.351599 0.359392 0.359392 0.359392 0.367126 0.367126 0.367126 0.374835 0.374835 0.374835 0.382562 0.382562 0.382562 0.390352 0.390352 0.390352 0.398256 0.398256 0.398256 0.406325 0.406325 0.406325 0.41461 0.41461 0.41461 0.423156 0.423156 0.423156 0.431994 0.431994 0.431994 0.441132 0.441132 0.441132 0.450548 0.450548 0.450548 0.460189 0.460189 0.460189 0.467051 0.467051 0.467051 0.5 0.5 0.5 0.532949 0.532949 0.532949 0.539811 0.539811 0.539811 0.549452 0.549452 0.549452 0.558868 0.558868 0.558868 0.568006 0.568006 0.568006 0.576844 0.576844 0.576844 0.58539 0.58539 0.58539 0.593675 0.593675 0.593675 0.601744 0.601744 0.601744 0.609648 0.609648 0.609648 0.617438 0.617438 0.617438 0.625165 0.625165 0.625165 0.632874 0.632874 0.632874 0.640608 0.640608 0.640608 0.648401 0.648401 0.648401 0.656287 0.656287 0.656287 0.664294 0.664294 0.664294 0.672444 0.672444 0.672444 0.680759 0.680759 0.680759 0.689257 0.689257 0.689257 0.697953 0.697953 0.697953 0.706861 0.706861 0.706861 0.715992 0.715992 0.715992 0.725357 0.725357 0.725357 0.734965 0.734965 0.734965 0.744824 0.744824 0.744824 0.75494 0.75494 0.75494 0.765319 0.765319 0.765319 0.777716 0.777716 0.777716 0.794089 0.794089 0.794089 0.802889 0.802889 0.802889 0.812862 0.812862 0.812862 0.824009 0.824009 0.824009 0.836328 0.836328 0.836328 0.849822 0.849822 0.849822 0.864488 0.864488 0.864488 0.880328 0.880328 0.880328 0.897341 0.897341 0.897341 0.915527 0.915527 0.915527 0.934887 0.934887 0.934887 1 1 1 1
  arc A286 (45.2631, 85.4069) -> (44.2745, 85.2932) centre (45.7832, 76.5321) ccw
  line L65 (48.6894, 80.7219) -> (48.2412, 79.6878)
  arc A287 (46.4062, 80.4833) -> (48.2412, 79.6878) centre (45.7832, 76.5321) ccw
  line L66 (46.8545, 81.5174) -> (46.4062, 80.4833)
  line L67 (48.6894, 80.7219) -> (46.8545, 81.5174)
  arc A288 (25.9058, 35.4989) -> (26.1558, 36.5892) centre (0.0409, 42.0024) ccw
  spline S84 degree 3 poles (26.6047, 39.6251) (26.4137, 39.5644) (26.1637, 39.4926) (25.8563, 39.419) (25.6922, 39.3833) (25.538, 39.3532) (25.3939, 39.3281) (25.26, 39.3077) (25.1365, 39.2915) (25.0234, 39.2791) (24.9208, 39.27) (24.829, 39.2638) (24.7478, 39.2601) (24.6774, 39.2582) (24.6178, 39.258) (24.5514, 39.2589) (24.4924, 39.2627) (24.4373, 39.2649) (24.4003, 39.2657) (24.3643, 39.2658) (24.3291, 39.2653) (24.2946, 39.2641) (24.261, 39.2621) (24.228, 39.2595) (24.1956, 39.2561) (24.1638, 39.252) (24.1325, 39.247) (24.1015, 39.2411) (24.0708, 39.2342) (24.0402, 39.2262) (24.0096, 39.2169) (23.9787, 39.2061) (23.9474, 39.1934) (23.9155, 39.1783) (23.8829, 39.1605) (23.8493, 39.139) (23.815, 39.113) (23.7803, 39.0815) (23.746, 39.0432) (23.7136, 38.9974) (23.6855, 38.9438) (23.6647, 38.8859) (23.6371, 38.7432) (23.6148, 38.5161) (23.5704, 38.2924) (23.5555, 38.1477) (23.5587, 38.0863) (23.5701, 38.0268) (23.5878, 37.9736) (23.6095, 37.9271) (23.6337, 37.8868) (23.659, 37.852) (23.6849, 37.8218) (23.711, 37.7952) (23.7372, 37.7716) (23.7634, 37.7504) (23.7898, 37.7311) (23.8165, 37.7133) (23.8434, 37.6968) (23.8708, 37.6813) (23.8988, 37.6667) (23.9273, 37.6529) (23.9566, 37.6397) (23.9866, 37.6271) (24.0174, 37.615) (24.0491, 37.6034) (24.0817, 37.5923) (24.1152, 37.5816) (24.1498, 37.5713) (24.1853, 37.5614) (24.2387, 37.5475) (24.2963, 37.5341) (24.3601, 37.5157) (24.4171, 37.4982) (24.484, 37.4761) (24.5606, 37.449) (24.6467, 37.4165) (24.7422, 37.3781) (24.8469, 37.3335) (24.9605, 37.2822) (25.0827, 37.224) (25.2134, 37.1583) (25.3523, 37.0848) (25.4991, 37.0031) (25.7719, 36.8437) (25.9905, 36.7026) (26.1558, 36.5892) knots 0 0 0 0 0.085622 0.111078 0.134991 0.157361 0.178189 0.197474 0.215216 0.231415 0.246072 0.259186 0.270757 0.280785 0.28927 0.296213 0.309142 0.314525 0.319779 0.32491 0.329923 0.334826 0.339627 0.344336 0.348964 0.353525 0.358035 0.362514 0.366985 0.371475 0.37602 0.380661 0.385447 0.39044 0.395711 0.401345 0.407436 0.41408 0.421363 0.429333 0.437971 0.447155 0.455484 0.5 0.544516 0.552845 0.562029 0.570667 0.578637 0.58592 0.592564 0.598655 0.604289 0.60956 0.614553 0.619339 0.62398 0.628525 0.633015 0.637486 0.641965 0.646475 0.651036 0.655664 0.660373 0.665174 0.670077 0.67509 0.680221 0.685475 0.690858 0.703787 0.71073 0.719215 0.729243 0.740814 0.753928 0.768585 0.784784 0.802526 0.821811 0.842639 0.865009 0.888922 0.914378 1 1 1 1
  arc A289 (26.6047, 39.6251) -> (26.6811, 40.7411) centre (0.0409, 42.0024) ccw
  spline S85 degree 3 poles (26.6496, 43.8099) (26.4704, 43.72) (26.2347, 43.61) (25.9426, 43.4892) (25.7861, 43.4283) (25.6385, 43.3744) (25.5001, 43.3271) (25.3711, 43.286) (25.2516, 43.2507) (25.1418, 43.2208) (25.042, 43.1958) (24.9522, 43.1752) (24.8726, 43.1588) (24.8033, 43.146) (24.7445, 43.1364) (24.6788, 43.1269) (24.6199, 43.1214) (24.5651, 43.115) (24.5286, 43.11) (24.4929, 43.1045) (24.4582, 43.0985) (24.4244, 43.0919) (24.3914, 43.0847) (24.3593, 43.077) (24.3278, 43.0686) (24.2971, 43.0595) (24.2669, 43.0497) (24.2372, 43.039) (24.208, 43.0274) (24.179, 43.0147) (24.1502, 43.0008) (24.1214, 42.9852) (24.0925, 42.9677) (24.0634, 42.9479) (24.0339, 42.9252) (24.0041, 42.8987) (23.9743, 42.8677) (23.9449, 42.8311) (23.917, 42.7879) (23.8923, 42.7376) (23.8728, 42.6803) (23.8614, 42.6199) (23.8564, 42.4746) (23.87, 42.2468) (23.8611, 42.0189) (23.869, 41.8737) (23.8817, 41.8135) (23.9023, 41.7566) (23.9281, 41.7068) (23.9569, 41.6642) (23.987, 41.6282) (24.0175, 41.5978) (24.0478, 41.572) (24.0777, 41.5498) (24.1073, 41.5306) (24.1365, 41.5137) (24.1656, 41.4988) (24.1947, 41.4854) (24.2239, 41.4733) (24.2534, 41.4623) (24.2833, 41.4523) (24.3136, 41.4431) (24.3446, 41.4346) (24.3762, 41.4269) (24.4085, 41.4198) (24.4416, 41.4133) (24.4756, 41.4074) (24.5104, 41.4021) (24.5461, 41.3973) (24.5828, 41.3931) (24.6377, 41.3878) (24.6967, 41.3835) (24.7626, 41.3753) (24.8216, 41.367) (24.8911, 41.3556) (24.971, 41.3408) (25.0612, 41.3221) (25.1615, 41.2992) (25.2719, 41.2715) (25.3921, 41.2386) (25.5219, 41.2002) (25.6613, 41.1557) (25.81, 41.1049) (25.9677, 41.0472) (26.2621, 40.9324) (26.5001, 40.8273) (26.6811, 40.7411) knots 0 0 0 0 0.085622 0.111078 0.134991 0.157361 0.178189 0.197474 0.215216 0.231415 0.246072 0.259186 0.270757 0.280785 0.28927 0.296213 0.309142 0.314525 0.319779 0.32491 0.329923 0.334826 0.339627 0.344336 0.348964 0.353525 0.358035 0.362514 0.366985 0.371475 0.37602 0.380661 0.385447 0.39044 0.395711 0.401345 0.407436 0.41408 0.421363 0.429333 0.437971 0.447155 0.455484 0.5 0.544516 0.552845 0.562029 0.570667 0.578637 0.58592 0.592564 0.598655 0.604289 0.60956 0.614553 0.619339 0.62398 0.628525 0.633015 0.637486 0.641965 0.646475 0.651036 0.655664 0.660373 0.665174 0.670077 0.67509 0.680221 0.685475 0.690858 0.703787 0.71073 0.719215 0.729243 0.740814 0.753928 0.768585 0.784784 0.802526 0.821811 0.842639 0.865009 0.888922 0.914378 1 1 1 1
  arc A290 (26.6496, 43.8099) -> (26.5504, 44.924) centre (0.0409, 42.0024) ccw
  spline S86 degree 3 poles (26.0392, 47.9502) (25.8764, 47.8333) (25.6607, 47.6878) (25.3911, 47.5228) (25.2461, 47.4382) (25.1088, 47.3619) (24.9794, 47.2935) (24.8584, 47.2327) (24.7459, 47.1792) (24.6422, 47.1324) (24.5475, 47.0921) (24.462, 47.0578) (24.386, 47.0291) (24.3196, 47.0056) (24.263, 46.987) (24.1996, 46.9673) (24.1423, 46.9527) (24.0891, 46.9377) (24.0538, 46.9271) (24.0195, 46.9161) (23.9861, 46.9047) (23.9538, 46.8929) (23.9223, 46.8807) (23.8918, 46.868) (23.862, 46.8548) (23.8331, 46.841) (23.8048, 46.8266) (23.7772, 46.8114) (23.7501, 46.7954) (23.7235, 46.7783) (23.6972, 46.76) (23.6712, 46.7401) (23.6454, 46.7184) (23.6197, 46.6942) (23.5942, 46.6671) (23.5689, 46.6364) (23.5443, 46.601) (23.521, 46.5603) (23.5002, 46.5133) (23.4836, 46.4598) (23.4734, 46.4001) (23.4715, 46.3386) (23.4894, 46.1943) (23.5384, 45.9715) (23.5653, 45.745) (23.5958, 45.6028) (23.6178, 45.5453) (23.647, 45.4923) (23.6803, 45.4472) (23.7153, 45.4097) (23.7507, 45.3788) (23.7856, 45.3536) (23.8195, 45.3328) (23.8526, 45.3156) (23.8848, 45.3012) (23.9163, 45.2892) (23.9474, 45.2789) (23.9782, 45.2703) (24.009, 45.2629) (24.0398, 45.2566) (24.0709, 45.2514) (24.1023, 45.2471) (24.1342, 45.2436) (24.1666, 45.2408) (24.1997, 45.2389) (24.2334, 45.2377) (24.2678, 45.2371) (24.303, 45.2373) (24.3391, 45.2382) (24.376, 45.2398) (24.431, 45.2431) (24.49, 45.2481) (24.5563, 45.2504) (24.6159, 45.2513) (24.6863, 45.251) (24.7676, 45.2489) (24.8596, 45.2445) (24.9623, 45.2376) (25.0756, 45.2275) (25.1994, 45.2138) (25.3337, 45.1962) (25.4783, 45.1741) (25.6331, 45.1471) (25.7979, 45.1148) (26.1067, 45.0475) (26.3582, 44.9809) (26.5504, 44.924) knots 0 0 0 0 0.085622 0.111078 0.134991 0.157361 0.178189 0.197474 0.215216 0.231415 0.246072 0.259186 0.270757 0.280785 0.28927 0.296213 0.309142 0.314525 0.319779 0.32491 0.329923 0.334826 0.339627 0.344336 0.348964 0.353525 0.358035 0.362514 0.366985 0.371475 0.37602 0.380661 0.385447 0.39044 0.395711 0.401345 0.407436 0.41408 0.421363 0.429333 0.437971 0.447155 0.455484 0.5 0.544516 0.552845 0.562029 0.570667 0.578637 0.58592 0.592564 0.598655 0.604289 0.60956 0.614553 0.619339 0.62398 0.628525 0.633015 0.637486 0.641965 0.646475 0.651036 0.655664 0.660373 0.665174 0.670077 0.67509 0.680221 0.685475 0.690858 0.703787 0.71073 0.719215 0.729243 0.740814 0.753928 0.768585 0.784784 0.802526 0.821811 0.842639 0.865009 0.888922 0.914378 1 1 1 1
  arc A291 (26.0392, 47.9502) -> (25.767, 49.0351) centre (0.0409, 42.0024) ccw
  spline S87 degree 3 poles (24.7887, 51.944) (24.6461, 51.8031) (24.4559, 51.6256) (24.2154, 51.4205) (24.0854, 51.3142) (23.9617, 51.2174) (23.8447, 51.1296) (23.7347, 51.0506) (23.6319, 50.9801) (23.5368, 50.9177) (23.4496, 50.8631) (23.3705, 50.8158) (23.2999, 50.7756) (23.238, 50.742) (23.185, 50.7148) (23.1254, 50.6854) (23.0711, 50.662) (23.021, 50.639) (22.9878, 50.6229) (22.9556, 50.6067) (22.9244, 50.5902) (22.8943, 50.5735) (22.8652, 50.5565) (22.837, 50.5392) (22.8097, 50.5215) (22.7832, 50.5033) (22.7576, 50.4847) (22.7327, 50.4654) (22.7084, 50.4453) (22.6848, 50.4243) (22.6617, 50.4021) (22.6391, 50.3784) (22.617, 50.3529) (22.5954, 50.325) (22.5744, 50.2942) (22.5543, 50.2599) (22.5355, 50.2212) (22.5189, 50.1773) (22.5057, 50.1276) (22.4977, 50.0721) (22.4969, 50.0116) (22.5047, 49.9506) (22.5449, 49.8108) (22.6282, 49.5984) (22.6902, 49.3789) (22.7426, 49.2433) (22.7733, 49.19) (22.8104, 49.1422) (22.8504, 49.1028) (22.8909, 49.0712) (22.9306, 49.0463) (22.969, 49.0268) (23.0058, 49.0116) (23.0411, 48.9998) (23.0752, 48.9906) (23.1082, 48.9836) (23.1405, 48.9784) (23.1723, 48.9746) (23.2038, 48.9722) (23.2353, 48.9708) (23.2668, 48.9705) (23.2985, 48.9711) (23.3305, 48.9727) (23.363, 48.9751) (23.3959, 48.9783) (23.4294, 48.9824) (23.4635, 48.9872) (23.4983, 48.9929) (23.5337, 48.9994) (23.5699, 49.0068) (23.6238, 49.0187) (23.6812, 49.0328) (23.7464, 49.0454) (23.8051, 49.0557) (23.8747, 49.0664) (23.9553, 49.077) (24.0468, 49.0871) (24.1493, 49.0963) (24.2628, 49.1041) (24.3873, 49.1099) (24.5227, 49.1135) (24.669, 49.1143) (24.8261, 49.1119) (24.9939, 49.1057) (25.3094, 49.0876) (25.5682, 49.0611) (25.767, 49.0351) knots 0 0 0 0 0.085622 0.111078 0.134991 0.157361 0.178189 0.197474 0.215216 0.231415 0.246072 0.259186 0.270757 0.280785 0.28927 0.296213 0.309142 0.314525 0.319779 0.32491 0.329923 0.334826 0.339627 0.344336 0.348964 0.353525 0.358035 0.362514 0.366985 0.371475 0.37602 0.380661 0.385447 0.39044 0.395711 0.401345 0.407436 0.41408 0.421363 0.429333 0.437971 0.447155 0.455484 0.5 0.544516 0.552845 0.562029 0.570667 0.578637 0.58592 0.592564 0.598655 0.604289 0.60956 0.614553 0.619339 0.62398 0.628525 0.633015 0.637486 0.641965 0.646475 0.651036 0.655664 0.660373 0.665174 0.670077 0.67509 0.680221 0.685475 0.690858 0.703787 0.71073 0.719215 0.729243 0.740814 0.753928 0.768585 0.784784 0.802526 0.821811 0.842639 0.865009 0.888922 0.914378 1 1 1 1
  arc A292 (24.7887, 51.944) -> (24.3501, 52.9729) centre (0.0409, 42.0024) ccw
  spline S88 degree 3 poles (22.9288, 55.693) (22.81, 55.5315) (22.6499, 55.3265) (22.4445, 55.0863) (22.3327, 54.961) (22.2257, 54.846) (22.1238, 54.741) (22.0275, 54.6458) (21.937, 54.5601) (21.8528, 54.4835) (21.7752, 54.4159) (21.7045, 54.3569) (21.6411, 54.3061) (21.5852, 54.2633) (21.5371, 54.228) (21.4829, 54.1897) (21.4329, 54.1581) (21.387, 54.1275) (21.3567, 54.1065) (21.3275, 54.0854) (21.2993, 54.0643) (21.2721, 54.043) (21.246, 54.0217) (21.2209, 54.0001) (21.1967, 53.9784) (21.1734, 53.9563) (21.151, 53.9339) (21.1294, 53.9109) (21.1086, 53.8873) (21.0885, 53.8629) (21.0692, 53.8373) (21.0506, 53.8104) (21.0328, 53.7817) (21.0158, 53.7508) (20.9999, 53.7172) (20.9854, 53.6801) (20.9729, 53.6389) (20.9633, 53.593) (20.9581, 53.5419) (20.9588, 53.4858) (20.9676, 53.4259) (20.9848, 53.3668) (21.0463, 53.2351) (21.1618, 53.0384) (21.2574, 52.8312) (21.3304, 52.7054) (21.369, 52.6576) (21.4132, 52.6162) (21.4588, 52.5836) (21.5037, 52.5587) (21.5469, 52.5403) (21.5879, 52.527) (21.6266, 52.5178) (21.6633, 52.5116) (21.6984, 52.5079) (21.7321, 52.5062) (21.7648, 52.5061) (21.7968, 52.5073) (21.8283, 52.5098) (21.8596, 52.5134) (21.8908, 52.518) (21.922, 52.5236) (21.9534, 52.5302) (21.9851, 52.5376) (22.0171, 52.5459) (22.0496, 52.5552) (22.0825, 52.5653) (22.1159, 52.5764) (22.1499, 52.5884) (22.1845, 52.6013) (22.2359, 52.6215) (22.2904, 52.6444) (22.3528, 52.6671) (22.4091, 52.6864) (22.4762, 52.7078) (22.5541, 52.7309) (22.643, 52.7552) (22.7428, 52.7803) (22.8537, 52.8058) (22.9757, 52.8311) (23.1089, 52.8558) (23.2532, 52.8794) (23.4088, 52.9016) (23.5755, 52.9218) (23.8899, 52.9532) (24.1497, 52.9676) (24.3501, 52.9729) knots 0 0 0 0 0.085622 0.111078 0.134991 0.157361 0.178189 0.197474 0.215216 0.231415 0.246072 0.259186 0.270757 0.280785 0.28927 0.296213 0.309142 0.314525 0.319779 0.32491 0.329923 0.334826 0.339627 0.344336 0.348964 0.353525 0.358035 0.362514 0.366985 0.371475 0.37602 0.380661 0.385447 0.39044 0.395711 0.401345 0.407436 0.41408 0.421363 0.429333 0.437971 0.447155 0.455484 0.5 0.544516 0.552845 0.562029 0.570667 0.578637 0.58592 0.592564 0.598655 0.604289 0.60956 0.614553 0.619339 0.62398 0.628525 0.633015 0.637486 0.641965 0.646475 0.651036 0.655664 0.660373 0.665174 0.670077 0.67509 0.680221 0.685475 0.690858 0.703787 0.71073 0.719215 0.729243 0.740814 0.753928 0.768585 0.784784 0.802526 0.821811 0.842639 0.865009 0.888922 0.914378 1 1 1 1
  arc A293 (22.9288, 55.693) -> (22.3346, 56.6407) centre (0.0409, 42.0024) ccw
  spline S89 degree 3 poles (20.5053, 59.1049) (20.4133, 58.9269) (20.2872, 58.6993) (20.1219, 58.4299) (20.0311, 58.2886) (19.9434, 58.1583) (19.8592, 58.0387) (19.7789, 57.9296) (19.703, 57.8308) (19.6318, 57.742) (19.5657, 57.6631) (19.5052, 57.5937) (19.4504, 57.5337) (19.4019, 57.4826) (19.36, 57.4403) (19.3124, 57.394) (19.268, 57.3549) (19.2274, 57.3175) (19.2008, 57.292) (19.1752, 57.2666) (19.1507, 57.2413) (19.1272, 57.2161) (19.1047, 57.1909) (19.0833, 57.1657) (19.0628, 57.1404) (19.0432, 57.115) (19.0246, 57.0893) (19.0068, 57.0633) (18.99, 57.0367) (18.974, 57.0094) (18.9589, 56.9812) (18.9448, 56.9517) (18.9317, 56.9206) (18.9197, 56.8874) (18.9092, 56.8517) (18.9007, 56.8128) (18.8948, 56.7701) (18.8926, 56.7232) (18.8954, 56.672) (18.9049, 56.6167) (18.9229, 56.5589) (18.9491, 56.5033) (19.0305, 56.3828) (19.1754, 56.2065) (19.3022, 56.0169) (19.3939, 55.9041) (19.4396, 55.8629) (19.4897, 55.8289) (19.5398, 55.8038) (19.5881, 55.7863) (19.6336, 55.7748) (19.6762, 55.7682) (19.7159, 55.7651) (19.7531, 55.7647) (19.7883, 55.7666) (19.8219, 55.7701) (19.8542, 55.7751) (19.8856, 55.7814) (19.9164, 55.7888) (19.9467, 55.7972) (19.9768, 55.8067) (20.0067, 55.8171) (20.0367, 55.8284) (20.0668, 55.8407) (20.0972, 55.854) (20.1278, 55.8682) (20.1587, 55.8834) (20.19, 55.8995) (20.2217, 55.9167) (20.2539, 55.9348) (20.3014, 55.9628) (20.3516, 55.994) (20.4097, 56.0261) (20.4624, 56.054) (20.5253, 56.0857) (20.5986, 56.1207) (20.6826, 56.1586) (20.7773, 56.199) (20.8828, 56.2415) (20.9994, 56.2855) (21.127, 56.3308) (21.2659, 56.3767) (21.416, 56.423) (21.5776, 56.469) (21.8832, 56.5492) (22.1376, 56.604) (22.3346, 56.6407) knots 0 0 0 0 0.085622 0.111078 0.134991 0.157361 0.178189 0.197474 0.215216 0.231415 0.246072 0.259186 0.270757 0.280785 0.28927 0.296213 0.309142 0.314525 0.319779 0.32491 0.329923 0.334826 0.339627 0.344336 0.348964 0.353525 0.358035 0.362514 0.366985 0.371475 0.37602 0.380661 0.385447 0.39044 0.395711 0.401345 0.407436 0.41408 0.421363 0.429333 0.437971 0.447155 0.455484 0.5 0.544516 0.552845 0.562029 0.570667 0.578637 0.58592 0.592564 0.598655 0.604289 0.60956 0.614553 0.619339 0.62398 0.628525 0.633015 0.637486 0.641965 0.646475 0.651036 0.655664 0.660373 0.665174 0.670077 0.67509 0.680221 0.685475 0.690858 0.703787 0.71073 0.719215 0.729243 0.740814 0.753928 0.768585 0.784784 0.802526 0.821811 0.842639 0.865009 0.888922 0.914378 1 1 1 1